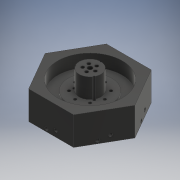
# Autodesk Inventor part: AC05
Saved by Autodesk Inventor 2017 (Build 210142000, 142)
## iProperties
Created: 2019-09-07
Part Number: AC05
Material: ABS Plastic
Document SubType Name: Modeling
Designer: Dell
Density: 1.06 g/cm^3
Appearance: Smooth - Black
Author: Dell
Autodesk Inventor part; units mm, degrees
ref_plane "YZ Plane" through (0, 0, 0) normal (1, 0, 0) x (0, 1, 0)
ref_plane "XZ Plane" through (0, 0, 0) normal (0, 1, 0) x (-1, 0, 0)
ref_plane "XY Plane" through (0, 0, 0) normal (0, 0, 1) x (1, 0, 0)
sketch "Sketch1" plane through (0, 0, 0) normal (0, 0, 1) x (1, 0, 0)
  circle A0 centre (0, 0) radius 3.5
  line L0 (77.9423, 0) -> (38.9711, -67.5)
  line L1 (38.9711, -67.5) -> (-38.9711, -67.5)
  line L2 (-38.9711, -67.5) -> (-77.9423, 0)
  line L3 (-77.9423, 0) -> (-38.9711, 67.5)
  line L4 (-38.9711, 67.5) -> (38.9711, 67.5)
  line L5 (38.9711, 67.5) -> (77.9423, 0)
  circle A1 centre (22.5, 0) radius 2.25
  circle A2 centre (54, 0) radius 2
  circle A3 centre (15.9099, 15.9099) radius 2.25
  circle A4 centre (0, 22.5) radius 2.25
  circle A5 centre (-15.9099, 15.9099) radius 2.25
  circle A6 centre (-22.5, 0) radius 2.25
  circle A7 centre (-15.9099, -15.9099) radius 2.25
  circle A8 centre (0, -22.5) radius 2.25
  circle A9 centre (15.9099, -15.9099) radius 2.25
  circle A10 centre (46.7654, 27) radius 2
  circle A11 centre (27, 46.7654) radius 2
  circle A12 centre (0, 54) radius 2
  circle A13 centre (-27, 46.7654) radius 2
  circle A14 centre (-46.7654, 27) radius 2
  circle A15 centre (-54, 0) radius 2
  circle A16 centre (-46.7654, -27) radius 2
  circle A17 centre (-27, -46.7654) radius 2
  circle A18 centre (0, -54) radius 2
  circle A19 centre (27, -46.7654) radius 2
  circle A20 centre (46.7654, -27) radius 2
  dimension "d0" = 7
  dimension "d1" = 135
  dimension "d2" = 22.5
  dimension "d3" = 4.5
  dimension "d4" = 4
  dimension "d5" = 54
  dimension "d8" = 360
  dimension "d12" = 360
  constraints: 21 centre point, 12 end point, 3 horizontal alignment, 2 coincident, 55 other
  measures "d0" diameter of A0
  measures "d1" distance between parallel lines of L1 L4
  measures "d2" distance of point (0, 0) A1.centre
  measures "d3" diameter of A1
  measures "d4" diameter of A2
  measures "d5" distance of point (0, 0) A2.centre
extrude "Extrusion1" add sketch "Sketch1" along normal blind 30
sketch "Sketch2" plane through (0, 0, 30) normal (0, 0, 1) x (1, 0, 0)
  circle A0 centre (0, 0) radius 3.5 projected
  circle A1 centre (0, 0) radius 49
  dimension "d16" = 98
  constraints: 1 centre point, 1 coincident
  measures "d16" diameter of A1
extrude "Extrusion2" cut sketch "Sketch2" against normal blind 15
sketch "Sketch3" plane through (0, 0, 15) normal (0, 0, 1) x (1, 0, 0)
  circle A0 centre (0, 0) radius 33
  dimension "d19" = 66
  constraints: 1 centre point, 1 coincident
  measures "d19" diameter of A0
extrude "Extrusion3" cut sketch "Sketch3" against normal blind 3
sketch "Sketch4" plane through (0, 0, 12) normal (0, 0, 1) x (1, 0, 0)
  circle A0 centre (0, 0) radius 16.5
  circle A1 centre (0, 0) radius 3.5 projected
  dimension "d22" = 33
  constraints: 1 centre point, 1 coincident
  measures "d22" diameter of A0
extrude "Extrusion4" add sketch "Sketch4" along normal blind 33
sketch "Sketch5" plane through (0, 0, 45) normal (0, 0, 1) x (1, 0, 0)
  circle A0 centre (8, 0) radius 2.5
  circle A1 centre (2.4721, 7.6085) radius 2.5
  circle A2 centre (-6.4721, 4.7023) radius 2.5
  circle A3 centre (-6.4721, -4.7023) radius 2.5
  circle A4 centre (2.4721, -7.6085) radius 2.5
  point P0 (0, 0)
  dimension "d25" = 5
  dimension "d26" = 8
  dimension "d29" = 360
  constraints: 5 centre point, 1 horizontal alignment, 11 other
  measures "d25" diameter of A0
  measures "d26" distance of point (0, 0) A0.centre
extrude "Extrusion5" cut sketch "Sketch5" against normal through all
sketch "Sketch6" plane through (0, 0, 0) normal (0, 0, -1) x (-1, 0, 0)
  circle A0 centre (0, 0) radius 17.5
  dimension "d33" = 35
  constraints: 1 centre point, 1 coincident
  measures "d33" diameter of A0
extrude "Extrusion6" cut sketch "Sketch6" against normal blind 5
sketch "Sketch10" plane through (0, 0, 0) normal (0, 0, -1) x (-1, 0, 0)
  circle A0 centre (22.5, 0) radius 2.25 projected
  circle A1 centre (0, 0) radius 3.5 projected
  circle A2 centre (0, 0) radius 20.25
  circle A3 centre (0, 0) radius 24.75
  circle A4 centre (0, 0) radius 16
  circle A5 centre (0, 0) radius 29
  line L0 (29, 0) -> (16, 0)
  dimension "d38" = 13
  constraints: 3 coincident, 2 centre point, 2 end point, 2 horizontal alignment, 2 tangent, 1 horizontal, 1 midpoint, 4 other
  measures "d38" distance of L0.start L0.end
extrude "Extrusion7" cut sketch "Sketch10" against normal blind 5 contours L0 A0 | A2 | A3 | A0 L0 | A5
sketch "Sketch11" plane through (0, 0, 12) normal (0, 0, 1) x (1, 0, 0)
  circle A0 centre (0, 0) radius 16.5 projected
  circle A1 centre (15.9099, -15.9099) radius 2.25 projected
  circle A2 centre (0, -22.5) radius 2.25 projected
  circle A3 centre (-15.9099, -15.9099) radius 2.25 projected
  circle A4 centre (-22.5, 0) radius 2.25 projected
  circle A5 centre (-15.9099, 15.9099) radius 2.25 projected
  circle A6 centre (0, 22.5) radius 2.25 projected
  circle A7 centre (15.9099, 15.9099) radius 2.25 projected
  circle A8 centre (22.5, 0) radius 2.25 projected
  circle A9 centre (0, 0) radius 33 projected
extrude "Extrusion8" add sketch "Sketch11" along normal up to surface (3 mm away) from surface at 0
sketch "Sketch12" plane through (0, 0, 30) normal (0, 0, 1) x (1, 0, 0)
  circle A0 centre (0, 0) radius 49 projected
  circle A1 centre (46.7654, -27) radius 2 projected
  circle A2 centre (27, -46.7654) radius 2 projected
  circle A3 centre (0, -54) radius 2 projected
  circle A4 centre (-27, -46.7654) radius 2 projected
  circle A5 centre (-46.7654, -27) radius 2 projected
  circle A6 centre (-54, 0) radius 2 projected
  circle A7 centre (-46.7654, 27) radius 2 projected
  circle A8 centre (-27, 46.7654) radius 2 projected
  circle A9 centre (0, 54) radius 2 projected
  circle A10 centre (27, 46.7654) radius 2 projected
  circle A11 centre (46.7654, 27) radius 2 projected
  circle A12 centre (54, 0) radius 2 projected
  line L0 (38.9711, -67.5) -> (77.9423, 0) projected
  line L1 (77.9423, 0) -> (38.9711, 67.5) projected
  line L2 (38.9711, 67.5) -> (-38.9711, 67.5) projected
  line L3 (-38.9711, 67.5) -> (-77.9423, 0) projected
  line L4 (-77.9423, 0) -> (-38.9711, -67.5) projected
  line L5 (-38.9711, -67.5) -> (38.9711, -67.5) projected
extrude "Extrusion9" cut sketch "Sketch12" against normal blind 1
sketch "Sketch14" plane through (0, 0, 15) normal (0, 0, 1) x (1, 0, 0)
  circle A0 centre (0, 0) radius 3.5 projected
  circle A1 centre (0, 0) radius 33
  circle A2 centre (15.9099, -15.9099) radius 2.25 projected
  circle A3 centre (0, -22.5) radius 2.25 projected
  circle A4 centre (-15.9099, -15.9099) radius 2.25 projected
  circle A5 centre (-22.5, 0) radius 2.25 projected
  circle A6 centre (-15.9099, 15.9099) radius 2.25 projected
  circle A7 centre (0, 22.5) radius 2.25 projected
  circle A8 centre (15.9099, 15.9099) radius 2.25 projected
  circle A9 centre (22.5, 0) radius 2.25 projected
  circle A10 centre (0, 0) radius 16.5 projected
  circle A11 centre (0, 0) radius 49 projected
  dimension "d45" = 66
  constraints: 1 centre point, 1 coincident
  measures "d45" diameter of A1
extrude "Extrusion10" cut sketch "Sketch14" against normal blind 4 contours A11
sketch "Sketch15" plane through (0, 0, 29) normal (0, 0, 1) x (1, 0, 0)
  circle A0 centre (0, 0) radius 49 construction
  circle A1 centre (54, 0) radius 2 construction
  circle A2 centre (46.7654, 27) radius 2 construction
  circle A3 centre (27, 46.7654) radius 2 construction
  circle A4 centre (0, 54) radius 2 construction
  circle A5 centre (-27, 46.7654) radius 2 construction
  circle A6 centre (-46.7654, 27) radius 2 construction
  circle A7 centre (-54, 0) radius 2 construction
  circle A8 centre (-46.7654, -27) radius 2 construction
  circle A9 centre (-27, -46.7654) radius 2 construction
  circle A10 centre (0, -54) radius 2 construction
  circle A11 centre (27, -46.7654) radius 2 construction
  circle A12 centre (46.7654, -27) radius 2 construction
  line L0 (77.9423, 0) -> (38.9711, -67.5) projected
  line L1 (38.9711, 67.5) -> (77.9423, 0) projected
  line L2 (-38.9711, 67.5) -> (38.9711, 67.5) projected
  line L3 (-77.9423, 0) -> (-38.9711, 67.5) projected
  line L4 (-38.9711, -67.5) -> (-77.9423, 0) projected
  line L5 (38.9711, -67.5) -> (-38.9711, -67.5) projected
  line L6 (36.0844, 62.5) -> (72.1688, 0)
  line L7 (72.1688, 0) -> (36.0844, -62.5)
  line L8 (36.0844, -62.5) -> (-36.0844, -62.5)
  line L9 (-36.0844, -62.5) -> (-72.1688, 0)
  line L10 (-72.1688, 0) -> (-36.0844, 62.5)
  line L11 (-36.0844, 62.5) -> (36.0844, 62.5)
  dimension "d48" = 5
  constraints: 12 end point, 5 other
  measures "d48" distance between parallel lines of L2 L11
extrude "Extrusion11" add sketch "Sketch15" along normal blind 0.8
sketch "Sketch16" plane through (0, 0, 0) normal (0, 0, -1) x (-1, 0, 0)
  circle A0 centre (0, 0) radius 29 projected
  circle A1 centre (-46.7654, -27) radius 2 projected
  circle A2 centre (-27, -46.7654) radius 2 projected
  circle A3 centre (0, -54) radius 2 projected
  circle A4 centre (27, -46.7654) radius 2 projected
  circle A5 centre (46.7654, -27) radius 2 projected
  circle A6 centre (54, 0) radius 2 projected
  circle A7 centre (46.7654, 27) radius 2 projected
  circle A8 centre (27, 46.7654) radius 2 projected
  circle A9 centre (0, 54) radius 2 projected
  circle A10 centre (-27, 46.7654) radius 2 projected
  circle A11 centre (-46.7654, 27) radius 2 projected
  circle A12 centre (-54, 0) radius 2 projected
  line L0 (-77.9423, 0) -> (-38.9711, -67.5) projected
  line L1 (-38.9711, -67.5) -> (38.9711, -67.5) projected
  line L2 (38.9711, -67.5) -> (77.9423, 0) projected
  line L3 (77.9423, 0) -> (38.9711, 67.5) projected
  line L4 (38.9711, 67.5) -> (-38.9711, 67.5) projected
  line L5 (-38.9711, 67.5) -> (-77.9423, 0) projected
  line L6 (68.1273, 0) -> (34.0637, -59)
  line L7 (34.0637, -59) -> (-34.0637, -59)
  line L8 (-34.0637, -59) -> (-68.1273, 0)
  line L9 (-68.1273, 0) -> (-34.0637, 59)
  line L10 (-34.0637, 59) -> (34.0637, 59)
  line L11 (34.0637, 59) -> (68.1273, 0)
  dimension "d51" = 118
  constraints: 12 end point, 5 other
  measures "d51" distance between parallel lines of L9 L6
extrude "Extrusion12" cut sketch "Sketch16" along normal through all both and the other way through all contours L5 L4 L3 L2 L1 L0
sketch "Sketch17" plane through (0, 0, 0) normal (0, 0, -1) x (-1, 0, 0)
  circle A0 centre (0, -54) radius 2 projected
  circle A1 centre (0, -54) radius 2
  circle A2 centre (27, -46.7654) radius 2
  circle A3 centre (46.7654, -27) radius 2
  circle A4 centre (54, 0) radius 2
  circle A5 centre (46.7654, 27) radius 2
  circle A6 centre (27, 46.7654) radius 2
  circle A7 centre (0, 54) radius 2
  circle A8 centre (-27, 46.7654) radius 2
  circle A9 centre (-46.7654, 27) radius 2
  circle A10 centre (-54, 0) radius 2
  circle A11 centre (-46.7654, -27) radius 2
  circle A12 centre (-27, -46.7654) radius 2
  point P0 (0, 0)
  dimension "d56" = 360
  constraints: 12 centre point, 1 coincident, 1 concentric, 25 other
extrude "Extrusion13" add sketch "Sketch17" along normal up to surface (29 mm away) from surface at -29
sketch "Sketch18" plane through (0, 0, 0) normal (0, 0, -1) x (-1, 0, 0)
  line L0 (-46.188, 0) -> (-23.094, 40)
  line L1 (-23.094, 40) -> (23.094, 40)
  line L2 (23.094, 40) -> (46.188, 0)
  line L3 (46.188, 0) -> (23.094, -40)
  line L4 (23.094, -40) -> (-23.094, -40)
  line L5 (-23.094, -40) -> (-46.188, 0)
  line L6 (-19.0526, -33) -> (19.0526, -33)
  line L7 (19.0526, -33) -> (38.1051, 0)
  line L8 (38.1051, 0) -> (19.0526, 33)
  line L9 (19.0526, 33) -> (-19.0526, 33)
  line L10 (-19.0526, 33) -> (-38.1051, 0)
  line L11 (-38.1051, 0) -> (-19.0526, -33)
  line L12 (-34.0637, -59) -> (34.0637, -59) projected
  line L13 (34.0637, -59) -> (68.1273, 0) projected
  line L14 (68.1273, 0) -> (34.0637, 59) projected
  line L15 (34.0637, 59) -> (-34.0637, 59) projected
  line L16 (-34.0637, 59) -> (-68.1273, 0) projected
  line L17 (-68.1273, 0) -> (-34.0637, -59) projected
  circle A0 centre (0, 0) radius 29 projected
  dimension "d60" = 80
  dimension "d61" = 7
  constraints: 24 end point, 1 coincident, 1 horizontal alignment, 18 other
  measures "d60" distance between parallel lines of L1 L4
  measures "d61" distance between parallel lines of L4 L6
extrude "Extrusion14" add sketch "Sketch18" along normal blind 13 contours L0 L1 L2 L3 L4 L5 | L17 L16 L15 L14 L13 L12
sketch "Sketch19" plane through (68.1273, 0, 29) normal (0.8660254, 0.5, 0) x (0, 0, -1)
  line L0 (29, 15.0111) -> (29, 53.1162) projected
  line L1 (29, 15.0111) -> (42, 15.0111) projected
  line L2 (42, 53.1162) -> (42, 15.0111) projected
  line L3 (29, 53.1162) -> (42, 53.1162) projected
  line L4 (38, 26.9926) -> (33, 41.1347) construction
  circle A0 centre (38, 26.9926) radius 2.5
  circle A1 centre (33, 41.1347) radius 2.5
  point P0 (29, 34.0637)
  point P1 (35.5, 15.0111)
  point P2 (35.5, 34.0637)
  point P3 (29, 34.0637)
  dimension "d64" = 15
  dimension "d65" = 5
  dimension "d66" = 5
  dimension "d72" = 5
  constraints: 3 midpoint, 2 centre point, 2 coincident, 2 end point, 1 horizontal alignment, 1 vertical alignment
  measures "d64" distance of L4.start L4.end
  measures "d65" diameter of A0
  measures "d66" diameter of A1
  measures "d72" horizontal distance of L4.end L4.start
extrude "Extrusion15" cut sketch "Sketch19" against normal blind 30 contours A0 | A1
pattern_circular "Circular Pattern1" count 6 over 360 about axis through (0, 0, 0) along (0, 0, 1) of "Extrusion15"
sketch "Sketch21" plane through (0, 0, 5) normal (0, 0, -1) x (-1, 0, 0)
  circle A0 centre (0, 17.5) radius 2
  circle A1 centre (-15.1554, -8.75) radius 2
  circle A2 centre (15.1554, -8.75) radius 2
  point P0 (0, 0)
  dimension "d74" = 4
  dimension "d75" = 17.5
  dimension "d78" = 360
  constraints: 3 centre point, 1 vertical alignment, 7 other
  measures "d74" diameter of A0
  measures "d75" distance of A0.centre point (0, 0)
extrude "Extrusion16" cut sketch "Sketch21" against normal through all
sketch "Sketch22" plane through (0, 0, 5) normal (0, 0, -1) x (-1, 0, 0)
  circle A0 centre (-15.1554, -8.75) radius 2 projected
  circle A1 centre (0, 17.5) radius 2 projected
  circle A2 centre (15.1554, -8.75) radius 2 projected
  circle A3 centre (0, 0) radius 29 projected
  circle A4 centre (-22.5, 0) radius 2.25 projected
  circle A5 centre (-15.9099, 15.9099) radius 2.25 projected
  circle A6 centre (0, 22.5) radius 2.25 projected
  circle A7 centre (15.9099, 15.9099) radius 2.25 projected
  circle A8 centre (22.5, 0) radius 2.25 projected
  circle A9 centre (15.9099, -15.9099) radius 2.25 projected
  circle A10 centre (0, -22.5) radius 2.25 projected
  circle A11 centre (-15.9099, -15.9099) radius 2.25 projected
  circle A12 centre (6.4721, -4.7023) radius 2.5 projected
  circle A13 centre (-2.4721, 7.6085) radius 2.5 projected
  circle A14 centre (-8, 0) radius 2.5 projected
  circle A15 centre (6.4721, 4.7023) radius 2.5 projected
  circle A16 centre (-2.4721, -7.6085) radius 2.5 projected
  circle A17 centre (0, 0) radius 3.5 projected
extrude "Extrusion17" cut sketch "Sketch22" against normal blind 5
sketch "Sketch23" plane through (0, 0, 10) normal (0, 0, -1) x (-1, 0, 0)
  circle A0 centre (0, 0) radius 3.5 projected
  circle A1 centre (0, 0) radius 12
  dimension "d84" = 24
  constraints: 1 centre point, 1 coincident
  measures "d84" diameter of A1
extrude "Extrusion18" cut sketch "Sketch23" against normal blind 7
sketch "Sketch24" plane through (0, 0, 29) normal (0, 0, 1) x (1, 0, 0)
  line L0 (-34.0637, -59) -> (34.0637, -59) projected
  line L1 (34.0637, -59) -> (68.1273, 0) projected
  line L2 (68.1273, 0) -> (34.0637, 59) projected
  line L3 (34.0637, 59) -> (-34.0637, 59) projected
  line L4 (-34.0637, 59) -> (-68.1273, 0) projected
  line L5 (-68.1273, 0) -> (-34.0637, -59) projected
  circle A0 centre (0, 0) radius 49 projected
extrude "Extrusion19" add sketch "Sketch24" along normal blind 1
body "Solid1"
